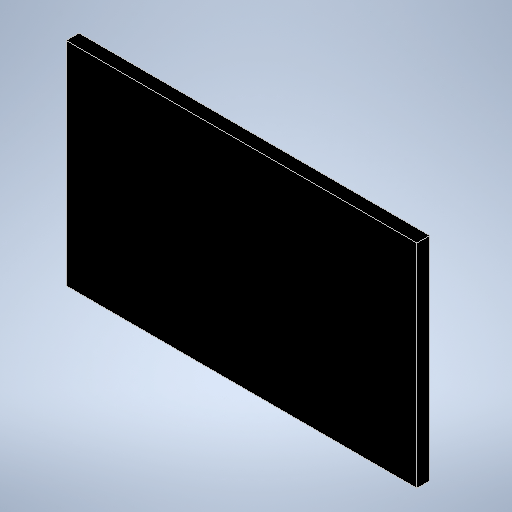
# Autodesk Inventor part: ShedMonitor
Saved by Autodesk Inventor 2025 (Build 290162010, 162A)
## iProperties
Created: 2024-08-20
Part Number: ShedMonitor
Material: Generic
Document SubType Name: Modeling
Designer: max_d
Density: 1 g/cm^3
Appearance: Default
Author: max_d
Autodesk Inventor part; units mm, degrees
ref_plane "YZ Plane" through (0, 0, 0) normal (1, 0, 0) x (0, 1, 0)
ref_plane "XZ Plane" through (0, 0, 0) normal (0, 1, 0) x (-1, 0, 0)
sketch "Sketch1" plane through (0, 0, 0) normal (0, 0, 1) x (1, 0, 0)
  line L0 (-272.5, -165) -> (272.5, -165)
  line L1 (272.5, -165) -> (272.5, 165)
  line L2 (272.5, 165) -> (-272.5, 165)
  line L3 (-272.5, 165) -> (-272.5, -165)
  line L4 (-272.5, -165) -> (272.5, 165) construction
  line L5 (272.5, -165) -> (-272.5, 165) construction
  point P0 (0, 0)
  dimension "d0" = 545
  dimension "d1" = 330
  constraints: 12 end point, 2 midpoint, 2 parallel, 1 horizontal, 1 perpendicular
  measures "d0" distance of L2.end L1.end
  measures "d1" distance of L1.end L0.end
extrude "Extrusion1" add sketch "Sketch1" along normal blind 20
sketch "Sketch2" plane through (0, 0, 0) normal (0, 0, -1) x (-1, 0, 0)
  line L0 (-205, -100) -> (205, -100)
  line L1 (205, -100) -> (205, 100)
  line L2 (205, 100) -> (-205, 100)
  line L3 (-205, 100) -> (-205, -100)
  line L4 (-205, -100) -> (205, 100) construction
  line L5 (205, -100) -> (-205, 100) construction
  point P0 (0, 0)
  dimension "d4" = 410
  dimension "d5" = 200
  constraints: 12 end point, 2 midpoint, 2 parallel, 1 horizontal, 1 perpendicular
  measures "d4" distance of L2.end L1.end
  measures "d5" distance of L1.end L0.end
ref_plane "Work Plane1" through (0, 0, -25) normal (0, 0, -1) x (-1, 0, 0)
sketch "Sketch3" plane through (0, 0, -25) normal (0, 0, -1) x (-1, 0, 0)
  line L0 (-175, -70) -> (175, -70)
  line L1 (175, -70) -> (175, 70)
  line L2 (175, 70) -> (-175, 70)
  line L3 (-175, 70) -> (-175, -70)
  line L4 (-175, -70) -> (175, 70) construction
  line L5 (175, -70) -> (-175, 70) construction
  point P0 (0, 0)
  dimension "d7" = 350
  dimension "d8" = 140
  constraints: 12 end point, 2 midpoint, 2 parallel, 1 horizontal, 1 perpendicular
  measures "d7" distance of L2.end L1.end
  measures "d8" distance of L0.end L1.end
loft "Loft1" add profiles "Sketch2", "Sketch3"
body "Solid1"
